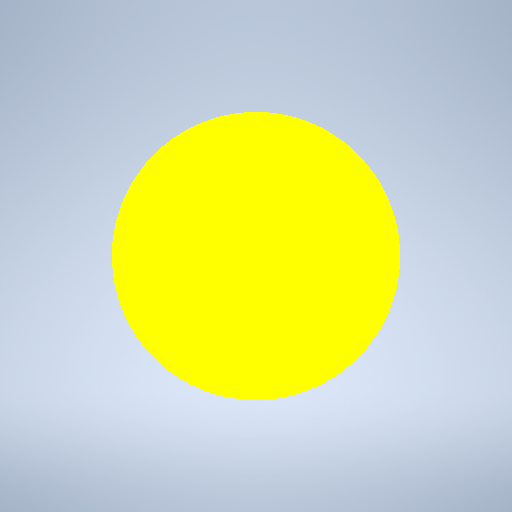
# Autodesk Inventor part: ボール2
Saved by Autodesk Inventor 2026.2 (Build 302298010, 298A)
## iProperties
Created: 2026-05-06
Part Number: ボール2
Material: 一般
Document SubType Name: Modeling
Designer: Yagis
Density: 1 g/cm^3
Appearance: 既定
Author: Yagis
Autodesk Inventor part; units mm, degrees
ref_plane "YZ Plane" through (0, 0, 0) normal (1, 0, 0) x (0, 1, 0)
ref_plane "XZ Plane" through (0, 0, 0) normal (0, 1, 0) x (-1, 0, 0)
ref_plane "XY Plane" through (0, 0, 0) normal (0, 0, 1) x (1, 0, 0)
sketch "スケッチ1" plane through (0, 0, 0) normal (0, 0, 1) x (1, 0, 0)
  circle A0 centre (0, 0) radius 32.5
  line L0 (0, 32.5) -> (0, -32.5)
  dimension "d0" = 65
  constraints: 2 end point, 2 point on circle, 1 centre point, 1 coincident
  measures "d0" diameter of A0
revolve "回転1" add sketch "スケッチ1" angle 360 about axis through (0, 32.5, 0) along (0, -1, 0) picked at (-8.9157, -6.154) contours L0 A0
